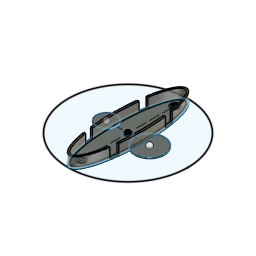
Cap_DualCircles (Autodesk Fusion 360 design; units mm, degrees)
Autodesk Fusion 360 part; units mm, degrees
sketch "Sketch1" plane through (0, 0, 0) normal (0, 0, 1) x (1, 0, 0)
  ellipse E0 centre (0, 0) end of major axis (0, -28.9) minor radius 6.85
  line L0 (0, 28.9) -> (0, -28.9) construction
  line L1 (-6.85, 0) -> (6.85, 0) construction
  ellipse E1 centre (0, 0) end of major axis (0, -29.9) minor radius 7.85
  circle A0 centre (0, 0) radius 2
  circle A1 centre (0, -23.9) radius 2
  circle A2 centre (0, 23.9) radius 2
  circle A3 centre (0, 0) radius 30.5
  circle A4 centre (11, 0) radius 7.5
  circle A5 centre (-11, 0) radius 5
  dimension "d1" = 57.8
  dimension "d2" = 13.7
  dimension "d3" = 4
  dimension "d4" = 4
  dimension "d5" = 4
  dimension "d6" = 5
  dimension "d7" = 5
  dimension "d24" = 61
  dimension "d25" = 15
  dimension "d26" = 10
  dimension "d27" = 11
  dimension "d28" = 11
  constraint coincident E0 L0.start
  constraint coincident E0 L0.end
  constraint coincident E0 L1.start
  constraint coincident E0 L1.end
  constraint coincident E0.centre E1.centre
  constraint vertical L0
  constraint concentric E1 A0
  constraint coincident L0 A1.centre
  constraint coincident L0 A2.centre
  measures "d1" distance of E0
  measures "d3" diameter of A0
  measures "d4" diameter of A1
  measures "d5" diameter of A2
  measures "d6" distance of L0.start A2.centre
  measures "d7" distance of L0.end A1.centre
  measures "d24" diameter of A3
  measures "d25" diameter of A4
  measures "d26" diameter of A5
  measures "d27" distance of E0.centre A4.centre
  measures "d28" distance of E0.centre A5.centre
extrude "Extrude1" add sketch "Sketch1" against normal blind 0.5 contours E0 A4 A5 | E0 A4 | E0 A5 makes body 1
extrude "Extrude2" add sketch "Sketch1" along normal blind 5 separate body contours E0 E1 A4 A5 | E0 E1 A4 | E0 E1 A5 | E0 E1 A4 A5 makes body 2
extrude "Extrude3" add sketch "Sketch1" against normal blind 0.5 contours E0 E1 A4 A5 | E0 E1 A4 | E0 E1 A5 | E0 E1 A4 A5 bodies 1 2
sketch "Sketch2" plane through (0, 0, 5) normal (0, 0, 1) x (-1, 0, 0)
  ellipse E0 centre (0, 0) end of major axis (0, 28.9) minor radius 6.85
  ellipse E1 centre (0, 0) end of major axis (0, 29.9) minor radius 7.85
  line L0 (10.7175, -15.9) -> (-9.5351, -15.9)
  line L1 (-9.5351, -15.9) -> (-9.5351, -11.9)
  line L2 (-9.5351, -11.9) -> (10.7175, -11.9)
  line L3 (10.7175, -11.9) -> (10.7175, -15.9)
  line L4 (12, 11.9) -> (-12, 11.9)
  line L5 (-12, 11.9) -> (-12, 15.9)
  line L6 (-12, 15.9) -> (12, 15.9)
  line L7 (12, 15.9) -> (12, 11.9)
  point P0 (0, -28.9)
  point P1 (0, 28.9)
  dimension "d18" = 4
  dimension "d19" = 13
  dimension "d20" = 4
  dimension "d21" = 13
  constraint horizontal L0
  constraint vertical L1
  constraint horizontal L2
  constraint vertical L3
  constraint coincident E0 P0
  constraint coincident E0 P1
  constraint horizontal L4
  constraint vertical L5
  constraint horizontal L6
  constraint vertical L7
  measures "d18" distance of L0.start L2.end
  measures "d19" distance of L0 P0
  measures "d20" distance of L4.start L6.end
  measures "d21" distance of P1 L6
extrude "Extrude4" cut sketch "Sketch2" against normal blind 5 contours E0 E1 L4 L6 | E0 E1 L4 L6 | E0 E1 L0 L2 | E0 E1 L0 L2 bodies 1
extrude "Extrude5" add sketch "Sketch1" against normal blind 0.5 contours E1 A4 bodies 1
extrude "Extrude6" add sketch "Sketch1" against normal blind 0.5 contours E1 A5 bodies 1
